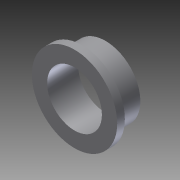
# Autodesk Inventor part: 276-2181-011 Rev1
Saved by Autodesk Inventor 2013 (Build 170138000, 138)
## iProperties
Category: Motors
Company: Autodesk Inc.
Created: 2012-01-23
Part Number: 276-2181-011 Rev1
Material: Generic
Document SubType Name: Modeling
Designer: Autodesk Inc.
Density: 1 g/cm^3
Catalog Web Link: http://www.vexrobotics.com/276-2181.html
Vendor: VEX
Author: Autodesk Inc.
Autodesk Inventor part; units mm, degrees
ref_plane "YZ Plane" through (0, 0, 0) normal (1, 0, 0) x (0, 1, 0)
ref_plane "XZ Plane" through (0, 0, 0) normal (0, 1, 0) x (-1, 0, 0)
ref_plane "XY Plane" through (0, 0, 0) normal (0, 0, 1) x (1, 0, 0)
sketch "Sketch1" plane through (0, 0, 0) normal (0, 0, 1) x (1, 0, 0)
  circle A0 centre (0, 0) radius 5.4991
  dimension "d0" = 10.9982
  constraints: 1 centre point, 1 coincident
  measures "d0" diameter of A0
extrude "Extrusion1" add sketch "Sketch1" against normal blind 0.9906
sketch "Sketch2" plane through (0, 0, -0.9906) normal (0, 0, -1) x (-1, 0, 0)
  circle A0 centre (0, 0) radius 5.4991 projected
  circle A1 centre (0, 0) radius 4.4958
  dimension "d3" = 8.9916
  constraints: 1 centre point, 1 coincident
  measures "d3" diameter of A1
extrude "Extrusion2" add sketch "Sketch2" along normal blind 2.9972 contours A1
sketch "Sketch3" plane through (0, 0, 0) normal (0, 0, 1) x (1, 0, 0)
  circle A0 centre (0, 0) radius 5.4991 projected
hole "Hole1" at (0, 0, 0) direction (0, 0, -1) diameter 7.0612 end through all
body "Solid1"
